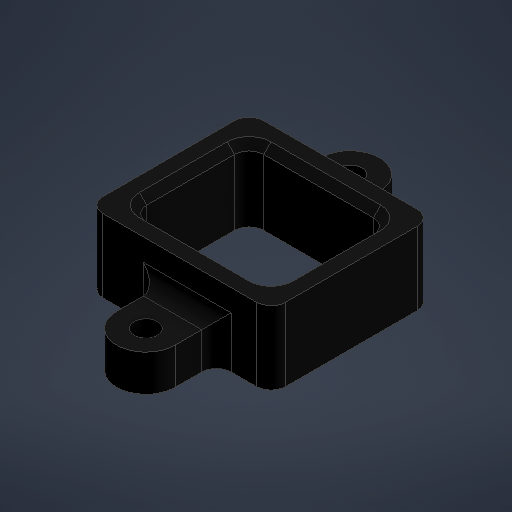
# Autodesk Inventor part: SchussAkkuHalterung
Saved by Autodesk Inventor 2025.2 (Build 292293000, 293)
## iProperties
Created: 2024-05-17
Part Number: SchussAkkuHalterung
Material: Generisch
Document SubType Name: Modeling
Designer: Fabian
Density: 1 g/cm^3
Appearance: Vorgabe
Author: Fabian
Autodesk Inventor part; units mm, degrees
ref_plane "YZ Plane" through (0, 0, 0) normal (1, 0, 0) x (0, 1, 0)
ref_plane "XZ Plane" through (0, 0, 0) normal (0, 1, 0) x (-1, 0, 0)
ref_plane "XY Plane" through (0, 0, 0) normal (0, 0, 1) x (1, 0, 0)
sketch "Skizze1" plane through (0, 0, 0) normal (0, 1, 0) x (-1, 0, 0)
  line L0 (19.0016, 59.2215) -> (57.3401, 24.0908)
  arc A0 (57.3401, 24.0908) -> (69.3003, 22.9246) centre (64.096, 31.4636) ccw
  arc A1 (75.2406, 20.5635) -> (69.3003, 22.9246) centre (71.3821, 19.509) ccw
  arc A2 (77.999, -0.3892) -> (75.2406, 20.5635) centre (0, 0) ccw
  arc A3 (72.8723, -4.2072) -> (77.999, -0.3892) centre (73.9991, -0.3692) ccw
  arc A4 (72.8723, -4.2072) -> (61.6214, -8.4293) centre (70.0553, -13.8022) ccw
  line L1 (61.6214, -8.4293) -> (37.5911, -46.1492)
  arc A5 (34.2176, -48) -> (37.5911, -46.1492) centre (34.2176, -44) ccw
  line L2 (34.2176, -48) -> (29, -48)
  arc A6 (29, -48) -> (25.0078, -51.75) centre (29, -52) ccw
  arc A7 (21.0156, -55.5) -> (25.0078, -51.75) centre (21.0156, -51.5) ccw
  line L3 (21.0156, -55.5) -> (-21.0156, -55.5)
  circle A8 centre (36.75, -68) radius 1.8
  circle A9 centre (36.75, -61) radius 1.8
  circle A10 centre (36.75, -54) radius 1.8
  line L4 (30.1812, 62.5407) -> (59.6723, 35.5171)
  arc A11 (59.6723, 35.5171) -> (68.1495, 35.8873) centre (63.7258, 39.9408) ccw
  line L5 (68.1495, 35.8873) -> (74.1043, 42.3858)
  arc A12 (77.3365, 41.9889) -> (74.1043, 42.3858) centre (75.5788, 41.0346) ccw
  arc A13 (85.5688, -20.542) -> (77.3365, 41.9889) centre (0, 0) ccw
  arc A14 (82.5495, -21.7619) -> (85.5688, -20.542) centre (83.6241, -20.0751) ccw
  line L6 (82.5495, -21.7619) -> (75.1157, -17.026)
  arc A15 (75.1157, -17.026) -> (66.8315, -18.8626) centre (71.8919, -22.0864) ccw
  line L7 (66.8315, -18.8626) -> (45.3395, -52.5983)
  arc A16 (45.3395, -52.5983) -> (47.1761, -60.8824) centre (50.3999, -55.8221) ccw
  line L8 (47.1761, -60.8824) -> (54.6099, -65.6183)
  arc A17 (54.7803, -68.8703) -> (54.6099, -65.6183) centre (53.5353, -67.3051) ccw
  arc A18 (44.8368, -75.7209) -> (54.7803, -68.8703) centre (0, 0) ccw
  arc A19 (43.8178, -76) -> (44.8368, -75.7209) centre (43.8178, -74) ccw
  line L9 (43.8178, -76) -> (35.75, -76)
  arc A20 (33.75, -74) -> (35.75, -76) centre (35.75, -74) ccw
  line L10 (33.75, -74) -> (33.75, -64)
  arc A21 (33.75, -64) -> (30.0179, -63) centre (31.75, -64) ccw
  arc A22 (28.2859, -64) -> (30.0179, -63) centre (28.2859, -62) ccw
  line L11 (28.2859, -64) -> (14.7321, -64)
  circle A23 centre (49.9686, 39.6617) radius 1.8
  circle A24 centre (55.4982, 34.5948) radius 1.8
  circle A25 centre (58.5312, -25.3775) radius 1.8
  circle A26 centre (54.5014, -31.7029) radius 1.8
  circle A27 centre (62.5609, -19.052) radius 1.8
  line L12 (37.1695, -45.8805) -> (61.1997, -8.1606)
  arc A28 (73.0131, -3.7275) -> (61.1997, -8.1606) centre (70.0553, -13.8022) ccw
  arc A29 (73.0131, -3.7275) -> (77.499, -0.3867) centre (73.9991, -0.3692) ccw
  arc A30 (77.499, -0.3867) -> (74.7582, 20.4317) centre (0, 0) ccw
  arc A31 (74.7582, 20.4317) -> (69.5605, 22.4976) centre (71.3821, 19.509) ccw
  arc A32 (57.0023, 23.7222) -> (69.5605, 22.4976) centre (64.096, 31.4636) ccw
  line L13 (57.0023, 23.7222) -> (18.6638, 58.8529)
  line L14 (-21.0156, -55) -> (21.0156, -55)
  arc A33 (21.0156, -55) -> (24.5088, -51.7188) centre (21.0156, -51.5) ccw
  arc A34 (29, -47.5) -> (24.5088, -51.7188) centre (29, -52) ccw
  line L15 (29, -47.5) -> (34.2176, -47.5)
  arc A35 (34.2176, -47.5) -> (37.1695, -45.8805) centre (34.2176, -44) ccw
  line L16 (47.604, 37.0813) -> (31.5682, 51.7754)
  line L17 (31.5682, 51.7754) -> (63.6398, 22.3872)
  line L18 (63.6398, 22.3872) -> (50.128, 7.6416)
  line L19 (47.3023, 7.5183) -> (18.1798, 34.2041)
  line L20 (18.0564, 37.0298) -> (31.5682, 51.7754)
  line L21 (58.5312, -25.3775) -> (55.5793, -23.4969)
  line L22 (55.5793, -23.4969) -> (67.2656, -5.1532)
  line L23 (67.2656, -5.1532) -> (43.893, -41.8407)
  line L24 (43.893, -41.8407) -> (27.0252, -31.0947)
  line L25 (26.413, -28.3333) -> (47.6364, 4.9806)
  line L26 (50.3977, 5.5928) -> (67.2656, -5.1532)
  arc A36 (50.3977, 5.5928) -> (47.6364, 4.9806) centre (49.3231, 3.906) ccw
  arc A37 (47.3023, 7.5183) -> (50.128, 7.6416) centre (48.6535, 8.9928) ccw
  arc A38 (26.413, -28.3333) -> (27.0252, -31.0947) centre (28.0998, -29.4079) ccw
  line L27 (81.0045, 17) -> (62.0045, 17)
  line L28 (62.0045, 17) -> (62.0045, 1)
  line L29 (62.0045, 1) -> (81.0045, 1)
  line L30 (81.0045, 1) -> (81.0045, 17)
  line L31 (81.0045, 17) -> (62.0045, 1) construction
  line L32 (62.0045, 17) -> (81.0045, 1) construction
  arc A39 (-37.5911, -46.1492) -> (-34.2176, -48) centre (-34.2176, -44) ccw
  line L33 (-37.5911, -46.1492) -> (-61.6214, -8.4293)
  arc A40 (-61.6214, -8.4293) -> (-72.8723, -4.2072) centre (-70.0553, -13.8022) ccw
  arc A41 (-77.999, -0.3892) -> (-72.8723, -4.2072) centre (-73.9991, -0.3692) ccw
  arc A42 (-75.2406, 20.5635) -> (-77.999, -0.3892) centre (0, 0) ccw
  arc A43 (-69.3003, 22.9246) -> (-75.2406, 20.5635) centre (-71.3821, 19.509) ccw
  arc A44 (-69.3003, 22.9246) -> (-57.3401, 24.0908) centre (-64.096, 31.4636) ccw
  line L34 (-57.3401, 24.0908) -> (-19.0016, 59.2215)
  arc A45 (-19.0016, 59.2215) -> (-16.7974, 71.0346) centre (-25.7575, 66.5943) ccw
  arc A46 (-13.9276, 76.7465) -> (-16.7974, 71.0346) centre (-13.2134, 72.8108) ccw
  arc A47 (13.9276, 76.7465) -> (-13.9276, 76.7465) centre (0, 0) ccw
  arc A48 (16.7974, 71.0346) -> (13.9276, 76.7465) centre (13.2134, 72.8108) ccw
  arc A49 (16.7974, 71.0346) -> (19.0016, 59.2215) centre (25.7575, 66.5943) ccw
  line L35 (19.0016, 59.2215) -> (57.3401, 24.0908)
  arc A50 (57.3401, 24.0908) -> (69.3003, 22.9246) centre (64.096, 31.4636) ccw
  arc A51 (75.2406, 20.5635) -> (69.3003, 22.9246) centre (71.3821, 19.509) ccw
  arc A52 (77.999, -0.3892) -> (75.2406, 20.5635) centre (0, 0) ccw
  arc A53 (72.8723, -4.2072) -> (77.999, -0.3892) centre (73.9991, -0.3692) ccw
  arc A54 (72.8723, -4.2072) -> (61.6214, -8.4293) centre (70.0553, -13.8022) ccw
  line L36 (61.6214, -8.4293) -> (37.5911, -46.1492)
  arc A55 (34.2176, -48) -> (37.5911, -46.1492) centre (34.2176, -44) ccw
  line L37 (34.2176, -48) -> (29, -48)
  arc A56 (29, -48) -> (25.0078, -51.75) centre (29, -52) ccw
  arc A57 (21.0156, -55.5) -> (25.0078, -51.75) centre (21.0156, -51.5) ccw
  line L38 (21.0156, -55.5) -> (-21.0156, -55.5)
  arc A58 (-25.0078, -51.75) -> (-21.0156, -55.5) centre (-21.0156, -51.5) ccw
  arc A59 (-25.0078, -51.75) -> (-29, -48) centre (-29, -52) ccw
  line L39 (-29, -48) -> (-34.2176, -48)
  circle A60 centre (-24.9586, 79.1585) radius 2.8
  circle A61 centre (-76.682, 31.7627) radius 2.8
  circle A62 centre (-82.2899, -10.8337) radius 2.8
  circle A63 centre (-36.75, -68) radius 1.8
  circle A64 centre (-36.75, -61) radius 1.8
  circle A65 centre (-36.75, -54) radius 1.8
  circle A66 centre (-49.9686, 39.6617) radius 1.8
  circle A67 centre (-55.4982, 34.5948) radius 1.8
  circle A68 centre (-44.439, 44.7287) radius 1.8
  circle A69 centre (-62.5609, -19.052) radius 1.8
  circle A70 centre (-54.5014, -31.7029) radius 1.8
  circle A71 centre (-58.5312, -25.3775) radius 1.8
  circle A72 centre (36.75, -68) radius 1.8
  circle A73 centre (36.75, -61) radius 1.8
  circle A74 centre (36.75, -54) radius 1.8
  circle A75 centre (82.2899, -10.8337) radius 2.8
  circle A76 centre (76.682, 31.7627) radius 2.8
  circle A77 centre (24.9586, 79.1585) radius 2.8
  arc A78 (29.8111, 71.018) -> (30.1812, 62.5407) centre (34.2347, 66.9644) ccw
  line L40 (30.1812, 62.5407) -> (59.6723, 35.5171)
  arc A79 (59.6723, 35.5171) -> (68.1495, 35.8873) centre (63.7258, 39.9408) ccw
  line L41 (68.1495, 35.8873) -> (74.1043, 42.3858)
  arc A80 (77.3365, 41.9889) -> (74.1043, 42.3858) centre (75.5788, 41.0346) ccw
  arc A81 (85.5688, -20.542) -> (77.3365, 41.9889) centre (0, 0) ccw
  arc A82 (82.5495, -21.7619) -> (85.5688, -20.542) centre (83.6241, -20.0751) ccw
  line L42 (82.5495, -21.7619) -> (75.1157, -17.026)
  arc A83 (75.1157, -17.026) -> (66.8315, -18.8626) centre (71.8919, -22.0864) ccw
  line L43 (66.8315, -18.8626) -> (45.3395, -52.5983)
  arc A84 (45.3395, -52.5983) -> (47.1761, -60.8824) centre (50.3999, -55.8221) ccw
  line L44 (47.1761, -60.8824) -> (54.6099, -65.6183)
  arc A85 (54.7803, -68.8703) -> (54.6099, -65.6183) centre (53.5353, -67.3051) ccw
  arc A86 (44.8368, -75.7209) -> (54.7803, -68.8703) centre (0, 0) ccw
  arc A87 (43.8178, -76) -> (44.8368, -75.7209) centre (43.8178, -74) ccw
  line L45 (43.8178, -76) -> (35.75, -76)
  arc A88 (33.75, -74) -> (35.75, -76) centre (35.75, -74) ccw
  line L46 (33.75, -74) -> (33.75, -64)
  arc A89 (33.75, -64) -> (30.0179, -63) centre (31.75, -64) ccw
  arc A90 (28.2859, -64) -> (30.0179, -63) centre (28.2859, -62) ccw
  line L47 (28.2859, -64) -> (14.7321, -64)
  arc A91 (13, -63) -> (14.7321, -64) centre (14.7321, -62) ccw
  line L48 (-14.7321, -64) -> (-28.2859, -64)
  arc A92 (-30.0179, -63) -> (-28.2859, -64) centre (-28.2859, -62) ccw
  arc A93 (-30.0179, -63) -> (-33.75, -64) centre (-31.75, -64) ccw
  line L49 (-33.75, -64) -> (-33.75, -74)
  arc A94 (-35.75, -76) -> (-33.75, -74) centre (-35.75, -74) ccw
  line L50 (-35.75, -76) -> (-43.8178, -76)
  arc A95 (-44.8368, -75.7209) -> (-43.8178, -76) centre (-43.8178, -74) ccw
  arc A96 (-54.7803, -68.8703) -> (-44.8368, -75.7209) centre (0, 0) ccw
  arc A97 (-54.6099, -65.6183) -> (-54.7803, -68.8703) centre (-53.5353, -67.3051) ccw
  line L51 (-54.6099, -65.6183) -> (-47.1761, -60.8824)
  arc A98 (-47.1761, -60.8824) -> (-45.3395, -52.5983) centre (-50.3999, -55.8221) ccw
  line L52 (-45.3395, -52.5983) -> (-66.8315, -18.8626)
  arc A99 (-66.8315, -18.8626) -> (-75.1157, -17.026) centre (-71.8919, -22.0864) ccw
  line L53 (-75.1157, -17.026) -> (-82.5495, -21.7619)
  arc A100 (-85.5688, -20.542) -> (-82.5495, -21.7619) centre (-83.6241, -20.0751) ccw
  arc A101 (-77.3365, 41.9889) -> (-85.5688, -20.542) centre (0, 0) ccw
  arc A102 (-74.1043, 42.3858) -> (-77.3365, 41.9889) centre (-75.5788, 41.0346) ccw
  line L54 (-74.1043, 42.3858) -> (-68.1495, 35.8873)
  arc A103 (-68.1495, 35.8873) -> (-59.6723, 35.5171) centre (-63.7258, 39.9408) ccw
  line L55 (-59.6723, 35.5171) -> (-30.1812, 62.5407)
  arc A104 (-30.1812, 62.5407) -> (-29.8111, 71.018) centre (-34.2347, 66.9644) ccw
  line L56 (-29.8111, 71.018) -> (-35.7659, 77.5165)
  arc A105 (-35.0888, 80.7018) -> (-35.7659, 77.5165) centre (-34.2913, 78.8676) ccw
  arc A106 (35.0888, 80.7018) -> (-35.0888, 80.7018) centre (0, 0) ccw
  arc A107 (35.7659, 77.5165) -> (35.0888, 80.7018) centre (34.2913, 78.8676) ccw
  line L57 (35.7659, 77.5165) -> (29.8111, 71.018)
  circle A108 centre (49.9686, 39.6617) radius 1.8
  circle A109 centre (55.4982, 34.5948) radius 1.8
  circle A110 centre (58.5312, -25.3775) radius 1.8
  circle A111 centre (54.5014, -31.7029) radius 1.8
  circle A112 centre (44.439, 44.7287) radius 1.8
  circle A113 centre (62.5609, -19.052) radius 1.8
  line L58 (37.1695, -45.8805) -> (61.1997, -8.1606)
  arc A114 (73.0131, -3.7275) -> (61.1997, -8.1606) centre (70.0553, -13.8022) ccw
  arc A115 (73.0131, -3.7275) -> (77.499, -0.3867) centre (73.9991, -0.3692) ccw
  arc A116 (77.499, -0.3867) -> (74.7582, 20.4317) centre (0, 0) ccw
  arc A117 (74.7582, 20.4317) -> (69.5605, 22.4976) centre (71.3821, 19.509) ccw
  arc A118 (57.0023, 23.7222) -> (69.5605, 22.4976) centre (64.096, 31.4636) ccw
  line L59 (57.0023, 23.7222) -> (18.6638, 58.8529)
  arc A119 (16.3494, 71.2566) -> (18.6638, 58.8529) centre (25.7575, 66.5943) ccw
  arc A120 (16.3494, 71.2566) -> (13.8384, 76.2545) centre (13.2134, 72.8108) ccw
  arc A121 (13.8384, 76.2545) -> (-13.8384, 76.2545) centre (0, 0) ccw
  arc A122 (-13.8384, 76.2545) -> (-16.3494, 71.2566) centre (-13.2134, 72.8108) ccw
  arc A123 (-18.6638, 58.8529) -> (-16.3494, 71.2566) centre (-25.7575, 66.5943) ccw
  line L60 (-18.6638, 58.8529) -> (-57.0023, 23.7222)
  arc A124 (-69.5605, 22.4976) -> (-57.0023, 23.7222) centre (-64.096, 31.4636) ccw
  arc A125 (-69.5605, 22.4976) -> (-74.7582, 20.4317) centre (-71.3821, 19.509) ccw
  arc A126 (-74.7582, 20.4317) -> (-77.499, -0.3867) centre (0, 0) ccw
  arc A127 (-77.499, -0.3867) -> (-73.0131, -3.7275) centre (-73.9991, -0.3692) ccw
  arc A128 (-61.1997, -8.1606) -> (-73.0131, -3.7275) centre (-70.0553, -13.8022) ccw
  line L61 (-61.1997, -8.1606) -> (-37.1695, -45.8805)
  arc A129 (-37.1695, -45.8805) -> (-34.2176, -47.5) centre (-34.2176, -44) ccw
  line L62 (-34.2176, -47.5) -> (-29, -47.5)
  arc A130 (-24.5088, -51.7188) -> (-29, -47.5) centre (-29, -52) ccw
  arc A131 (-24.5088, -51.7188) -> (-21.0156, -55) centre (-21.0156, -51.5) ccw
  line L63 (-21.0156, -55) -> (21.0156, -55)
  arc A132 (21.0156, -55) -> (24.5088, -51.7188) centre (21.0156, -51.5) ccw
  arc A133 (29, -47.5) -> (24.5088, -51.7188) centre (29, -52) ccw
  line L64 (29, -47.5) -> (34.2176, -47.5)
  arc A134 (34.2176, -47.5) -> (37.1695, -45.8805) centre (34.2176, -44) ccw
  circle A135 centre (16, 9) radius 2.1
  line L65 (-19, -53) -> (-19, 12)
  circle A136 centre (4, 47) radius 1.621
  circle A137 centre (-4, 47) radius 1.621
  arc A138 (7, 49.9161) -> (10.3333, 45.972) centre (11, 49.9161) ccw
  arc A139 (12, 44) -> (10.3333, 45.972) centre (10, 44) ccw
  line L66 (12, 44) -> (12, -5)
  line L67 (12, -5) -> (10, -5)
  arc A140 (8, -3) -> (10, -5) centre (10, -3) ccw
  line L68 (8, -3) -> (8, 1)
  arc A141 (8, 1) -> (6, 3) centre (6, 1) ccw
  line L69 (6, 3) -> (-6, 3)
  arc A142 (-6, 3) -> (-8, 1) centre (-6, 1) ccw
  line L70 (-8, 1) -> (-8, -3)
  arc A143 (-10, -5) -> (-8, -3) centre (-10, -3) ccw
  line L71 (-10, -5) -> (-12, -5)
  line L72 (-12, -5) -> (-12, 44)
  arc A144 (-10.3333, 45.972) -> (-12, 44) centre (-10, 44) ccw
  arc A145 (-10.3333, 45.972) -> (-7, 49.9161) centre (-11, 49.9161) ccw
  line L73 (-7, 49.9161) -> (-7, 54)
  arc A146 (-5, 56) -> (-7, 54) centre (-5, 54) ccw
  line L74 (-5, 56) -> (5, 56)
  arc A147 (7, 54) -> (5, 56) centre (5, 54) ccw
  line L75 (7, 54) -> (7, 49.9161)
  line L76 (-13, -63) -> (13, -63) construction
  line L77 (0, -63) -> (0, 88) construction
  arc A148 (35.0888, 80.7018) -> (-35.0888, 80.7018) centre (0, 0) ccw construction
  line L78 (0, 0) -> (88, 0) construction
  arc A149 (85.5688, -20.542) -> (77.3365, 41.9889) centre (0, 0) ccw construction
  circle A150 centre (0, 0) radius 75 construction
  line L79 (0, 0) -> (70.4769, 25.6515) construction
  line L80 (0, 0) -> (74.7146, -6.5367) construction
  circle A151 centre (0, 0) radius 78
  circle A152 centre (70.4769, 25.6515) radius 3
  circle A153 centre (74.7146, -6.5367) radius 3
  circle A154 centre (0, 0) radius 72
  arc A155 (29, -48) -> (25.0078, -51.75) centre (29, -52) ccw construction
  circle A156 centre (29, -52) radius 3.5
  line L81 (34.2176, -48) -> (29, -48) construction
  line L82 (29, -55.5) -> (21.0156, -55.5)
  circle A157 centre (29, -52) radius 4
  line L83 (32.5, -48) -> (29, -48)
  arc A158 (21.0156, -55.5) -> (25.0078, -51.75) centre (21.0156, -51.5) ccw
  arc A159 (21.0156, -55.5) -> (25.0078, -51.75) centre (21.0156, -51.5) ccw
  line L84 (32.5, -52) -> (32.5, -48)
  circle A160 centre (74.7146, -6.5367) radius 1.6
  circle A161 centre (70.4769, 25.6515) radius 1.6
  circle A162 centre (29, -52) radius 1.6
  line L85 (0, -55.5) -> (0, 88)
  line L86 (84.0045, -2) -> (59.0045, -2)
  line L87 (59.0045, -2) -> (59.0045, 20)
  line L88 (59.0045, 20) -> (84.0045, 20)
  line L89 (84.0045, 20) -> (84.0045, -2)
  circle A163 centre (82.2899, -10.8337) radius 4
  line L90 (74.7146, -6.5367) -> (74.7146, 9.8771) construction
  line L91 (78.7146, -6.5367) -> (78.7146, 9.8771)
  line L92 (70.7146, 9.8771) -> (70.7146, -6.5367)
  arc A164 (70.7146, -6.5367) -> (78.7146, -6.5367) centre (74.7146, -6.5367) ccw
  arc A165 (78.7146, 9.8771) -> (70.7146, 9.8771) centre (74.7146, 9.8771) ccw
  line L93 (70.4769, 25.6515) -> (70.4769, 13.0481) construction
  line L94 (66.4769, 25.6515) -> (66.4769, 13.0481)
  line L95 (74.4769, 13.0481) -> (74.4769, 25.6515)
  arc A166 (74.4769, 25.6515) -> (66.4769, 25.6515) centre (70.4769, 25.6515) ccw
  arc A167 (66.4769, 13.0481) -> (74.4769, 13.0481) centre (70.4769, 13.0481) ccw
  point P0 (0, 0)
  point P1 (0, 0)
  point P2 (216.3011, -305.5849)
  point P3 (183.0204, -305.5849)
  point P4 (184.3011, -305.5849)
  point P5 (215.0204, -305.5849)
  point P6 (48.7768, 6.1671)
  point P7 (25.3384, -30.0201)
  point P8 (0, 0)
  point P9 (0, 0)
  point P10 (357.611, -164.2236)
  point P11 (324.3303, -164.2236)
  point P12 (325.611, -164.2236)
  point P13 (356.3303, -164.2236)
  point P14 (0, -5)
  point P15 (0, 56)
  point P16 (496.1935, -138.8477)
  point P17 (490.2163, -138.3247)
  point P18 (494.6235, -171.8005)
  point P19 (500.2617, -169.7483)
  point P20 (538.9195, -97.1229)
  point P21 (542.9117, -93.3729)
  point P22 (414.2667, -82.5461)
  point P23 (408.6285, -84.5982)
  point P24 (409.3834, -86.7803)
  point P25 (361.9863, -164.7236)
  point P26 (373.4707, -157.2236)
  point P27 (412.861, -113.1957)
  point P28 (412.6967, -115.4989)
  point P29 (418.6738, -116.0218)
  point P30 (418.9697, -109.6128)
  point P31 (416.2112, -88.6601)
  point P32 (340.9707, -31.2236)
  point P33 (340.9707, -53.2236)
  point P34 (340.9707, -97.2236)
  point P35 (340.9707, -100.2236)
  point P36 (340.9707, -164.7236)
  point P37 (74.7146, 1.6702)
  point P38 (70.4769, 19.3498)
  point P39 (70.7146, -2)
  point P40 (78.7146, -2)
  point P41 (66.4769, 20)
  point P42 (74.4769, 20)
  dimension "d0" = 0.5
  dimension "d1" = 43.5
  dimension "d2" = 22
  dimension "d3" = 3.5
  dimension "d4" = 21.75
  dimension "d5" = 43.5
  dimension "d6" = 22
  dimension "d7" = 2
  dimension "d8" = 19
  dimension "d9" = 16
  dimension "d10" = 1
  dimension "d11" = 0.5
  dimension "d20" = 4.2
  dimension "d23" = 65
  dimension "d26" = 150
  dimension "d27" = 20
  dimension "d28" = 5
  dimension "d29" = 156
  dimension "d30" = 6
  dimension "d31" = 6
  dimension "d32" = 7
  dimension "d33" = 4
  dimension "d34" = 3.2
  dimension "d35" = 3.2
  dimension "d36" = 3.2
  dimension "d37" = 3
  dimension "d38" = 8
  dimension "d39" = 8
  dimension "d40" = 8
  constraints: 250 point on circle, 196 end point, 168 centre point, 16 tangent, 14 coincident, 11 parallel, 7 perpendicular, 7 point on line, 5 midpoint, 2 collinear, 2 equal radius, 1 concentric, 1 vertical, 40 other
  measures "d0" distance between parallel lines of L1 L12
  measures "d1" distance of L16.end L17.end
  measures "d2" distance of L17.end point (48.777, 6.167)
  measures "d3" distance of L21.start L21.end
  measures "d4" distance of L21.end L22.end
  measures "d5" distance of L22.end L23.end
  measures "d6" distance of L23.end point (25.338, -30.02)
  measures "d7" radius of A36
  measures "d8" distance of L29.end L28.end
  measures "d9" distance of L28.end L27.end
  measures "d10" distance from line of L29 point (0, 0)
  measures "d11" distance between parallel lines of L36 L58
  measures "d20" diameter of A135
  measures "d23" distance of L65.start L65.end
  measures "d26" diameter of A150
  measures "d27" angle of L78 L79
  measures "d28" angle of L78 L80
  measures "d29" diameter of A151
  measures "d30" diameter of A152
  measures "d31" diameter of A153
  measures "d32" diameter of A156
  measures "d33" distance of L84.start L83.start
  measures "d34" diameter of A160
  measures "d35" diameter of A161
  measures "d36" diameter of A162
  measures "d37" distance between parallel lines of L29 L86
  measures "d38" diameter of A163
  measures "d39" diameter of A165
  measures "d40" diameter of A167
extrude "Extrusion1" add sketch "Skizze1" along normal blind 10 contours L88 L94 L27 L28 L29 L92 L86 L26 L87 L18 | L18 L87 L88 | L88 A154 L27 L94 | L88 L95 L27 A154 | L26 L86 L87 | L88 A30 L27 L95 | L88 A2 L27 A30 | L92 L29 A154 L86 | L88 L89 L86 L91 L29 L30 L27 A2 | A154 L29 A30 A29 L86 | A29 A30 L29 A2 A3 L86 | A3 A151 L86 | L29 L91 L86 A151 A2
extrude "Extrusion2" add sketch "Skizze1" along normal blind 5 contours L94 A166 A154 A0 | A0 A154 A32 L94 | A166 A151 A152 A154 | A154 A152 A0 | A0 A152 A31 A32 A154 | A32 A154 L88 L94 | A152 A1 A0 | A166 L95 A151 | A0 A1 A152 A31 | A32 A31 A152 L95 L88 A154 | A151 L95 A1 A152 | A31 A152 | A1 L95 A31 A152 | L86 A154 A28 L92 | A28 A154 A4 L92 | L86 A29 A153 A28 A154 | A28 A29 A153 A4 A154 | A4 A154 A164 L92 | L86 A3 A153 A29 | A164 A154 A153 A151 | A151 L86 L91 A164 | A4 A153 A154 | A153 A3 A4 A29 | A29 A153 | L86 A151 A153 A3 | A153 A4 A3
fillet "Rundung1" radius 2 6 edges at (-70.4769, 5, 20) (-66.4769, 2.5, 20) (-74.4769, 2.5, 20) (-70.7146, 2.5, -2) (-74.7146, 5, -2) (-78.7146, 2.5, -2)
fillet "Rundung2" radius 2 8 edges at (-59.0045, 5, 20) (-59.0045, 5, -2) (-84.0045, 5, 20) (-84.0045, 5, -2) (-81.0045, 5, 1) (-81.0045, 5, 17) (-62.0045, 5, 1) (-62.0045, 5, 17)
chamfer "Fasen1" distance 1 angle 45 4 edges at (-71.5045, 10, 1) (-62.0045, 10, 9) (-71.5045, 10, 17) (-81.0045, 10, 9)
sketch "Skizze2" plane through (0, 5, 0) normal (0, 1, 0) x (1, 0, 0)
  circle A0 centre (-74.7146, 6.5367) radius 1.6 projected
  circle A1 centre (-74.7146, 6.5367) radius 3
  point P0 (0, 0)
  dimension "d50" = 6
  constraints: 1 centre point, 1 coincident
  measures "d50" diameter of A1
extrude "Extrusion3" cut sketch "Skizze2" along normal blind 10 contours A0 | A1
